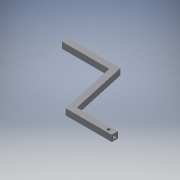
# Autodesk Inventor part: Arm Hatch
Saved by Autodesk Inventor 2017 (Build 210142000, 142)
## iProperties
Created: 2019-02-05
Part Number: Arm Hatch
Material: Generic
Document SubType Name: Modeling
Designer: S346795925
Density: 1 g/cm^3
Appearance: Default
Author: S346795925
Autodesk Inventor part; units mm, degrees
ref_plane "YZ Plane" through (0, 0, 0) normal (1, 0, 0) x (0, 1, 0)
ref_plane "XZ Plane" through (0, 0, 0) normal (0, 1, 0) x (-1, 0, 0)
ref_plane "XY Plane" through (0, 0, 0) normal (0, 0, 1) x (1, 0, 0)
sketch "Sketch1" plane through (0, 0, 0) normal (0, 1, 0) x (-1, 0, 0)
  line L0 (0, 0) -> (-101.6, 0)
  line L1 (-101.6, 0) -> (-127, 114.3)
  line L2 (-127, 114.3) -> (-215.9, 114.3)
  dimension "d0" = 101.6
  dimension "d2" = 114.3
  dimension "d3" = 25.4
  dimension "d4" = 88.9
  constraints: 6 end point, 1 horizontal, 1 parallel
  measures "d0" distance of L0.start L0.end
  measures "d2" distance between parallel lines of L0 L2
  measures "d3" horizontal distance of L0.end L1.end
  measures "d4" distance of L1.end L2.end
sketch "Sketch2" plane through (0, 0, 0) normal (1, 0, 0) x (0, 1, 0)
  line L0 (-6.35, 6.35) -> (6.35, 6.35)
  line L1 (6.35, 6.35) -> (6.35, -6.35)
  line L2 (6.35, -6.35) -> (-6.35, -6.35)
  line L3 (-6.35, -6.35) -> (-6.35, 6.35)
  line L4 (-6.35, 6.35) -> (6.35, -6.35) construction
  line L5 (6.35, 6.35) -> (-6.35, -6.35) construction
  line L6 (3.175, -3.175) -> (3.175, 3.175)
  line L7 (3.175, 3.175) -> (-3.175, 3.175)
  line L8 (-3.175, 3.175) -> (-3.175, -3.175)
  line L9 (-3.175, -3.175) -> (3.175, -3.175)
  point P0 (0, 0)
  dimension "d5" = 12.7
  dimension "d6" = 12.7
  dimension "d7" = 3.175
  constraints: 20 end point, 4 parallel, 2 midpoint, 2 perpendicular, 1 horizontal, 3 other
  measures "d5" distance of L1.end L2.end
  measures "d6" distance of L0.end L1.end
  measures "d7" distance between parallel lines of L1 L6
sweep "Sweep1" add profiles "Sketch2" path "Sketch1"
sketch "Sketch3" plane through (0, 6.35, 6.35) normal (0, 1, 0) x (1, 0, 0)
  circle A0 centre (203.2, -107.95) radius 3.175
  line L0 (215.9, -101.6) -> (215.9, -114.3) projected
  line L1 (121.9062, -114.3) -> (215.9, -114.3) projected
  point P0 (0, 6.35)
  dimension "d10" = 6.35
  dimension "d11" = 12.7
  dimension "d12" = 6.35
  constraints: 1 centre point
  measures "d10" diameter of A0
  measures "d11" distance from line of L0 A0.centre
  measures "d12" distance from line of L1 A0.centre
extrude "Extrusion1" cut sketch "Sketch3" against normal through all
body "Solid1"
